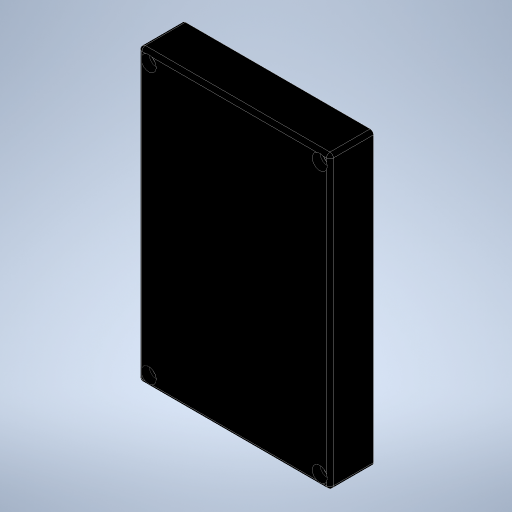
# Autodesk Inventor part: BatteryCase_Top
Saved by Autodesk Inventor 2024 (Build 280153000, 153)
## iProperties
Created: 2023-12-27
Part Number: BatteryCase_Top
Material: Generisch
Document SubType Name: Modeling
Designer: denni
Density: 1 g/cm^3
Appearance: Vorgabe(1)
Author: denni
Autodesk Inventor part; units mm, degrees
ref_plane "YZ Plane" through (0, 0, 0) normal (1, 0, 0) x (0, 1, 0)
ref_plane "XZ Plane" through (0, 0, 0) normal (0, 1, 0) x (-1, 0, 0)
ref_plane "XY Plane" through (0, 0, 0) normal (0, 0, 1) x (1, 0, 0)
sketch "Skizze1" plane through (0, 0, 0) normal (1, 0, 0) x (0, 1, 0)
  circle A0 centre (0, 0) radius 7.75
  line L0 (0, 0) -> (7.75, 0) construction
  circle A1 centre (17, 0) radius 7.75
  circle A2 centre (34, 0) radius 7.75
  circle A3 centre (51, 0) radius 7.75
  line L1 (66, 3.75) -> (-15, 3.75)
  line L2 (-15, 3.75) -> (-15, 9.75)
  line L3 (-15, 9.75) -> (66, 9.75)
  line L4 (66, 9.75) -> (66, 3.75)
  point P0 (24.75, 0)
  point P1 (41.75, 0)
  point P2 (58.75, 0)
  point P3 (66, 6.75)
  point P4 (-6.7823, 3.75)
  point P5 (6.7823, 3.75)
  point P6 (10.2177, 3.75)
  point P7 (23.7823, 3.75)
  point P8 (27.2177, 3.75)
  point P9 (40.7823, 3.75)
  point P10 (44.2177, 3.75)
  point P11 (57.7823, 3.75)
  dimension "d0" = 15.5
  dimension "d3" = 17
  dimension "a" = 9.75
  dimension "b" = 15
  dimension "d10" = 15
  dimension "d11" = 6
  constraints: 10 end point, 6 horizontal, 2 parallel, 1 coincident, 1 midpoint, 1 perpendicular, 18 other
  measures "d3" distance of L0.start point (17, 0)
  measures "a" distance from line of point (51, 0) L3
  measures "b" horizontal distance of point (66, 6.75) point (51, 0)
  measures "d10" distance from line of L2 point (0, 0)
  measures "d11" distance between parallel lines of L1 L3
extrude "Extrusion1" add sketch "Skizze1" along normal blind 10 contours A0 L1 L2 L3 L4 A3 A2 A1
sketch "Skizze2" plane through (0, -15, 9.75) normal (0, 0, 1) x (1, 0, 0)
  line L0 (0, 81) -> (10, 81) projected
  line L1 (10, 81) -> (-16, 81)
  line L2 (-16, 81) -> (-16, 0)
  line L3 (-16, 0) -> (10, 0)
  line L4 (10, 0) -> (10, 81)
  line L5 (0, 0) -> (10, 0) projected
  point P0 (0, 15)
  dimension "d14" = 26
  constraints: 8 end point, 2 parallel, 1 collinear, 1 horizontal, 1 perpendicular
  measures "d14" distance of L0.end L1.end
extrude "Extrusion2" add sketch "Skizze2" along normal blind 3
sketch "Skizze3" plane through (10, 0, 0) normal (1, 0, 0) x (0, 0, -1)
  line L0 (-12.75, 66) -> (-12.75, -15) projected
  line L1 (-12.75, 66) -> (17, 66)
  line L2 (17, 66) -> (17, -15)
  line L3 (17, -15) -> (-12.75, -15)
  line L4 (-12.75, -15) -> (-12.75, 66)
  line L5 (-3.75, -15) -> (-12.75, -15) construction
  circle A0 centre (17, 51) radius 2.5 construction
  point P0 (0, 0)
  point P1 (-12.75, -15)
  constraints: 8 end point, 2 parallel, 1 collinear, 1 horizontal, 1 perpendicular, 1 point on line
extrude "Extrusion3" add sketch "Skizze3" along normal blind 2
sketch "Skizze4" plane through (-16, -15, 9.75) normal (0, -1, 0) x (1, 0, 0)
  line L0 (0, 3) -> (28, 3) projected
  line L1 (28, -26.75) -> (28, 3) projected
  line L2 (0, 3) -> (28, 3)
  line L3 (28, 3) -> (28, -26.75)
  line L4 (28, -26.75) -> (0, -26.75)
  line L5 (0, -26.75) -> (0, 3)
  point P0 (16, -9.75)
  constraints: 8 end point, 2 parallel, 1 horizontal, 1 perpendicular
extrude "Extrusion4" add sketch "Skizze4" along normal blind 2
sketch "Skizze5" plane through (-16, 66, 9.75) normal (0, 1, 0) x (1, 0, 0)
  line L0 (0, 0) -> (0, 26.75) projected
  line L1 (28, -3) -> (0, -3)
  line L2 (0, -3) -> (0, 26.75)
  line L3 (0, 26.75) -> (28, 26.75)
  line L4 (28, 26.75) -> (28, -3)
  point P0 (16, 9.75)
  constraints: 8 end point, 2 parallel, 1 horizontal, 1 perpendicular
extrude "Extrusion5" add sketch "Skizze5" along normal blind 2
sketch "Skizze6" plane through (10, -15, -17) normal (0, 0, -1) x (-1, 0, 0)
  line L0 (-2, -2) -> (26, -2) projected
  line L1 (-2, -2) -> (4, -2)
  line L2 (4, -2) -> (4, 4)
  line L3 (4, 4) -> (-2, 4)
  line L4 (-2, 4) -> (-2, -2)
  line L5 (-2, 83) -> (26, 83) projected
  line L6 (-2, 83) -> (4, 83)
  line L7 (4, 83) -> (4, 77)
  line L8 (4, 77) -> (-2, 77)
  line L9 (-2, 77) -> (-2, 83)
  point P0 (10, 15)
  point P1 (4, 83)
  dimension "d23" = 6
  constraints: 16 end point, 4 parallel, 3 equal length, 2 horizontal, 2 perpendicular
  measures "d23" distance of L1.end L2.end
extrude "Extrusion6" add sketch "Skizze6" against normal up to surface (20.75 mm away)
fillet "Rundung1" radius 1 8 edges at (10, -11, -6.625) (6, -11, -6.625) (6, -15, -6.625) (12, -17, -2.125) (12, 68, -2.125) (10, 62, -6.625) (6, 62, -6.625) (6, 66, -6.625)
sketch "Skizze8" plane through (5, 66, 12.75) normal (0, 0, -1) x (-1, 0, 0)
  arc A0 (-6, 2) -> (-7, 1) centre (-6, 1) ccw construction
  arc A1 (-2, -4) -> (-1, -3) centre (-2, -3) ccw construction
  line L0 (-6, 1) -> (-2, -3) construction
  arc A2 (-7, -82) -> (-6, -83) centre (-6, -82) ccw construction
  line L1 (-6, -82) -> (-2, -78) construction
  point P0 (5, -66)
  point P1 (-4, -80)
  point P2 (-4, -1)
  constraints: 4 end point, 2 midpoint
hole "Bohrung2" at (9, 65, 12.75) at (9, -14, 12.75) direction (0, 0, -1) diameter 2.4 end through all counterbore diameter 4.4 counterbore depth 2.3 clearance for "Inbusschraube ISO 4762" size "M2" standard "ISO"
mirror "Spiegeln1" about plane through (-16, 66, 9.75) normal (-1, 0, 0) of "Extrusion1", "Extrusion2", "Extrusion3", "Extrusion4", "Extrusion5", "Extrusion6", "Rundung1", "Bohrung2"
sketch "Skizze7" plane through (0, -15, 9.75) normal (0, 0, -1) x (-1, 0, 0)
  line L0 (0, 81) -> (0, 0) projected
  line L1 (32, 0) -> (0, 0) projected
  line L2 (32, 81) -> (32, 0) projected
  line L3 (0, 81) -> (32, 81) projected
  point P0 (0, 15)
extrude "Extrusion7" add sketch "Skizze7" along normal blind 1
sketch "Skizze9" plane through (12, -16, -17) normal (0, 0, -1) x (-1, 0, 0)
  circle A0 centre (3, 81) radius 2.2 projected
  circle A1 centre (53, 2) radius 1.2 projected
  circle A2 centre (53, 81) radius 1.2 projected
  line L0 (49, 1) -> (7, 1) projected
  arc A3 (6, 2) -> (7, 1) centre (7, 2) ccw projected
  line L1 (6, 2) -> (6, 4) projected
  arc A4 (6, 4) -> (5, 5) centre (5, 4) ccw projected
  line L2 (5, 5) -> (3, 5) projected
  arc A5 (2, 6) -> (3, 5) centre (3, 6) ccw projected
  line L3 (2, 6) -> (2, 77) projected
  arc A6 (3, 78) -> (2, 77) centre (3, 77) ccw projected
  line L4 (3, 78) -> (5, 78) projected
  arc A7 (5, 78) -> (6, 79) centre (5, 79) ccw projected
  line L5 (6, 79) -> (6, 81) projected
  arc A8 (7, 82) -> (6, 81) centre (7, 81) ccw projected
  line L6 (7, 82) -> (49, 82) projected
  arc A9 (50, 81) -> (49, 82) centre (49, 81) ccw projected
  line L7 (50, 79) -> (50, 81) projected
  arc A10 (50, 79) -> (51, 78) centre (51, 79) ccw projected
  line L8 (53, 78) -> (51, 78) projected
  arc A11 (54, 77) -> (53, 78) centre (53, 77) ccw projected
  line L9 (54, 6) -> (54, 77) projected
  arc A12 (53, 5) -> (54, 6) centre (53, 6) ccw projected
  line L10 (51, 5) -> (53, 5) projected
  arc A13 (51, 5) -> (50, 4) centre (51, 4) ccw projected
  line L11 (50, 2) -> (50, 4) projected
  arc A14 (49, 1) -> (50, 2) centre (49, 2) ccw projected
  circle A15 centre (3, 2) radius 1.2 projected
  circle A16 centre (3, 81) radius 1.2 projected
  line L12 (1, -1) -> (55, -1) projected
  arc A17 (55, -1) -> (56, 0) centre (55, 0) ccw projected
  line L13 (56, 83) -> (56, 0) projected
  arc A18 (56, 83) -> (55, 84) centre (55, 83) ccw projected
  line L14 (1, 84) -> (55, 84) projected
  arc A19 (1, 84) -> (0, 83) centre (1, 83) ccw projected
  line L15 (0, 83) -> (0, 0) projected
  arc A20 (0, 0) -> (1, -1) centre (1, 0) ccw projected
  point P0 (12, 16)
extrude "Extrusion8" cut sketch "Skizze9" against normal blind 17 contours A0 | A20 L15 A19 L14 A18 L13 A17 L12
fillet "Rundung2" radius 1 4 edges at (-44, 25.5, 12.75) (-16, -17, 12.75) (12, 25.5, 12.75) (-16, 68, 12.75)
equation "\"d10\" = b"
